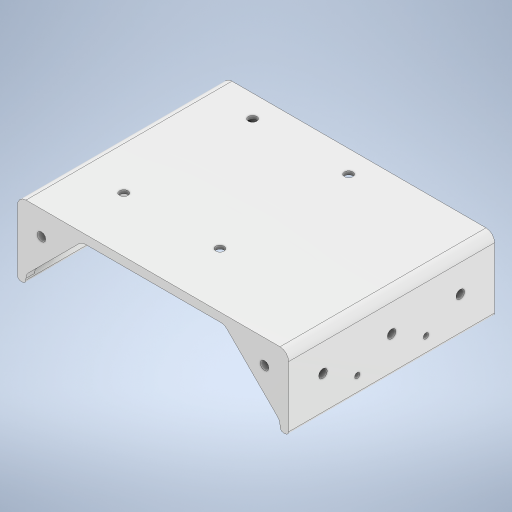
# Autodesk Inventor part: BP_BOX-Side-120-2
Saved by Autodesk Inventor 2024.3 (Build 283343000, 343)
## iProperties
Created: 2025-10-30
Part Number: BP_BOX-Side-120-2
Material: ABS プラスチック
Document SubType Name: Modeling
Designer: 佐藤智貴
Density: 1.06 g/cm^3
Appearance: 滑らか - 白
Mass: 64.4893 g
Surface Area: 354.929 cm^2
Volume: 60.8389 cm^3
Author: 佐藤智貴
Autodesk Inventor part; units mm, degrees
ref_plane "YZ Plane" through (0, 0, 0) normal (1, 0, 0) x (0, 1, 0)
ref_plane "XZ Plane" through (0, 0, 0) normal (0, 1, 0) x (-1, 0, 0)
ref_plane "XY Plane" through (0, 0, 0) normal (0, 0, 1) x (1, 0, 0)
sketch "スケッチ1" plane through (0, 0, 0) normal (0, 0, 1) x (1, 0, 0)
  line L0 (0, 0) -> (158, 0)
  line L1 (158, 0) -> (158, 250)
  line L2 (158, 250) -> (0, 250)
  line L3 (0, 250) -> (0, 0)
  line L4 (5, 245) -> (153, 245)
  line L5 (153, 245) -> (153, 5)
  line L6 (153, 5) -> (5, 5)
  line L7 (5, 5) -> (5, 245)
  line L8 (79, 250) -> (79, 0)
  line L9 (0, 125) -> (158, 125)
  line L10 (0, 245) -> (158, 245)
  line L11 (158, 245) -> (158, 3)
  line L12 (158, 3) -> (0, 3)
  line L13 (0, 3) -> (0, 245)
  point P0 (158, 245)
  point P1 (0, 3)
  point P2 (79, 3)
  point P3 (79, 5)
  point P4 (5, 125)
  point P5 (153, 125)
  point P6 (79, 245)
  point P7 (79, 245)
  point P8 (79, 125)
  point P9 (0, 3)
  dimension "d0" = 158
  dimension "d1" = 250
  dimension "d2" = 5
  dimension "d73" = 5
  constraints: 28 end point, 6 parallel, 4 midpoint, 3 perpendicular, 2 horizontal, 2 point on line, 3 other
  measures "d0" distance of L1.end L2.end
  measures "d1" distance between parallel lines of L0 L2
  measures "d2" distance between parallel lines of L2 L4
  measures "d73" distance between parallel lines of L2 L10
extrude "押し出し1" add sketch "スケッチ1" along normal blind 120 contours L3 L2 L8 L4 L10 | L10 L4 L8 L2 L1
sketch "スケッチ5" plane through (0, 0, 0) normal (0, 0, -1) x (-1, 0, 0)
  line L0 (0, 250) -> (0, 0) projected
  line L1 (0, 250) -> (-50, 250)
  line L2 (-50, 250) -> (-50, 200)
  line L3 (-50, 200) -> (0, 200)
  line L4 (0, 200) -> (0, 250)
  line L5 (-50, 250) -> (0, 200)
  line L6 (-46.2132, 253.7868) -> (3.7868, 203.7868)
  line L7 (0, 0) -> (-158, 0) projected
  line L8 (0, 125) -> (-79, 125)
  line L9 (-79, 125) -> (-79, 0)
  line L10 (-79, 0) -> (0, 0)
  line L11 (0, 0) -> (0, 125)
  line L12 (-46.2132, -3.7868) -> (3.7868, 46.2132)
  line L13 (-111.7868, 253.7868) -> (-161.7868, 203.7868)
  line L14 (-111.7868, -3.7868) -> (-161.7868, 46.2132)
  line L15 (0, 0) -> (-50, 0)
  line L16 (0, 50) -> (0, 0)
  line L17 (-158, 250) -> (-158, 0)
  line L18 (-158, 0) -> (0, 0)
  line L19 (-158, 250) -> (-108, 250)
  point P0 (0, 42.4264)
  point P1 (-42.4264, 0)
  point P2 (-158, 42.4264)
  point P3 (-115.5736, 0)
  point P4 (-42.4264, 250)
  point P5 (0, 207.5736)
  point P6 (-115.5736, 250)
  point P7 (-158, 207.5736)
  dimension "d29" = 50
  dimension "d30" = 50
  dimension "d31" = 30
  constraints: 36 end point, 12 symmetric about line, 5 parallel, 2 horizontal, 2 midpoint, 2 perpendicular
  measures "d29" distance of L2.end L3.end
  measures "d30" distance of L1.end L2.end
  measures "d31" distance from line of L0.start L6
extrude "押し出し3" add sketch "スケッチ5" against normal blind 5 contours L0 L6 L1 | L13 L17 L19
sketch "スケッチ6" plane through (0, 0, 120) normal (0, 0, 1) x (1, 0, 0)
  line L0 (0, 0) -> (50, 0)
  line L1 (50, 0) -> (50, 50)
  line L2 (50, 50) -> (0, 50)
  line L3 (0, 50) -> (0, 0)
  line L4 (50, 0) -> (0, 50)
  line L5 (46.2132, -3.7868) -> (-3.7868, 46.2132)
  line L6 (0, 250) -> (0, 0) projected
  line L7 (158, 250) -> (0, 250) projected
  line L8 (0, 125) -> (79, 125)
  line L9 (79, 125) -> (79, 250)
  line L10 (79, 250) -> (0, 250)
  line L11 (0, 250) -> (0, 125)
  line L12 (0, 250) -> (50, 250)
  line L13 (0, 200) -> (0, 250)
  line L14 (46.2132, 253.7868) -> (-3.7868, 203.7868)
  line L15 (158, 0) -> (108, 0)
  line L16 (158, 50) -> (158, 0)
  line L17 (111.7868, -3.7868) -> (161.7868, 46.2132)
  line L18 (158, 250) -> (158, 0)
  line L19 (158, 250) -> (108, 250)
  line L20 (111.7868, 253.7868) -> (161.7868, 203.7868)
  point P0 (158, 42.4264)
  point P1 (115.5736, 0)
  point P2 (158, 207.5736)
  point P3 (115.5736, 250)
  point P4 (0, 207.5736)
  point P5 (42.4264, 250)
  point P6 (42.4264, 0)
  point P7 (0, 42.4264)
  dimension "d34" = 50
  dimension "d35" = 50
  dimension "d37" = 30
  constraints: 38 end point, 14 symmetric about line, 5 parallel, 2 horizontal, 2 midpoint, 2 perpendicular
  measures "d34" distance of L1.end L2.end
  measures "d35" distance of L0.end L1.end
  measures "d37" distance from line of L5 L0.start
extrude "押し出し4" add sketch "スケッチ6" against normal blind 5 contours L6 L7 L14 | L18 L20 L7
sketch "スケッチ7" plane through (0, 0, 0) normal (0, 0, -1) x (-1, 0, 0)
  line L0 (0, 0) -> (-158, 0) projected
  line L1 (0, 124.7294) -> (-79, 124.7294)
  line L2 (-79, 124.7294) -> (-79, 0)
  line L3 (-79, 0) -> (0, 0)
  line L4 (0, 0) -> (0, 124.7294)
  line L5 (0, 250) -> (0, 0) projected
  line L6 (-158, 250) -> (0, 250) projected
  point P0 (-14, 236)
  point P1 (-14, 13.4587)
  point P2 (-144, 236)
  point P3 (-144, 13.4587)
  point P4 (0, 207.5736)
  dimension "d70" = 130
  dimension "d71" = 14
  dimension "d72" = 14
  constraints: 8 end point, 3 symmetric about line, 2 parallel, 1 horizontal, 1 midpoint, 1 perpendicular
  measures "d70" distance of point (-144, 236) point (-14, 236)
  measures "d71" distance from line of L5 point (-14, 236)
  measures "d72" distance from line of L6 point (-144, 236)
hole "穴2" at (14, 236, 0) at (14, 13.4587, 0) at (144, 236, 0) at (144, 13.4587, 0) direction (0, 0, 1) diameter 5 end through all
sketch "スケッチ8" plane through (158, 250, 120) normal (1, 0, 0) x (0, 0, -1)
  line L0 (120, 0) -> (0, 0) projected
  line L1 (120, -42.4264) -> (115, -42.4264) projected
  line L2 (0, 0) -> (120, 0)
  line L3 (120, 0) -> (120, -42.4264)
  line L4 (120, -42.4264) -> (0, -42.4264)
  line L5 (0, -42.4264) -> (0, 0)
  point P0 (120, -250)
  constraints: 8 end point, 2 parallel, 1 horizontal, 1 perpendicular
extrude "押し出し5" add sketch "スケッチ8" against normal blind 5
sketch "スケッチ9" plane through (0, 250, 0) normal (-1, 0, 0) x (0, 0, 1)
  line L0 (120, 0) -> (120, -42.4264) projected
  line L1 (0, 0) -> (0, -250) projected
  line L2 (120, 0) -> (0, 0)
  line L3 (0, 0) -> (0, -42.4264)
  line L4 (0, -42.4264) -> (120, -42.4264)
  line L5 (120, -42.4264) -> (120, 0)
  point P0 (120, -42.4264)
  point P1 (60, -250)
  constraints: 8 end point, 2 parallel, 1 horizontal, 1 perpendicular, 1 other
extrude "押し出し6" add sketch "スケッチ9" against normal blind 5
fillet "フィレット4" radius 5 12 edges at (0, 250, 60) (158, 250, 60) (120.5736, 245, 117.5) (120.5736, 245, 2.5) (153, 245, 60) (5, 245, 60) (37.4264, 245, 117.5) (37.4264, 245, 2.5) (153, 212.5736, 2.5) (153, 212.5736, 117.5) (5, 212.5736, 2.5) (5, 212.5736, 117.5)
fillet "フィレット6" radius 2 4 edges at (153, 207.5736, 60) (0, 207.5736, 60) (5, 207.5736, 60) (158, 207.5736, 60)
sketch "スケッチ12" plane through (37.4264, 245, 0) normal (0, -1, 0) x (1, 0, 0)
  line L0 (-27.4264, 5) -> (2.0711, 5) projected
  line L1 (2.0711, 0) -> (81.0761, 0) projected
  line L2 (81.0761, 5) -> (110.5736, 5) projected
  line L3 (110.5736, 115) -> (81.0761, 115) projected
  line L4 (2.0711, 120) -> (81.0761, 120) projected
  line L5 (2.0711, 115) -> (-27.4264, 115) projected
  line L6 (78.1472, 115) -> (78.1472, 110)
  line L7 (78.1472, 110) -> (108.5736, 110)
  line L8 (108.5736, 110) -> (108.5736, 10)
  line L9 (108.5736, 10) -> (76.1819, 10)
  line L10 (76.1819, 10) -> (76.1819, 5)
  line L11 (76.1819, 5) -> (3.0347, 5)
  line L12 (3.0347, 5) -> (3.0347, 10)
  line L13 (3.0347, 10) -> (-25.4264, 10)
  line L14 (-25.4264, 10) -> (-25.4264, 110)
  line L15 (-25.4264, 110) -> (3.0347, 110)
  line L16 (3.0347, 110) -> (3.0347, 115)
  line L17 (3.0347, 115) -> (78.1472, 115)
  line L18 (2.0711, 0) -> (2.0711, 5) projected
  line L19 (81.0761, 5) -> (81.0761, 0) projected
  line L20 (110.5736, 115) -> (110.5736, 5) projected
  line L21 (81.0761, 120) -> (81.0761, 115) projected
  line L22 (2.0711, 115) -> (2.0711, 120) projected
  line L23 (-27.4264, 5) -> (-27.4264, 115) projected
  line L24 (115.5736, 120) -> (115.5736, 0) projected
  line L25 (-32.4264, 0) -> (-32.4264, 120) projected
  point P0 (-37.4264, 0)
  dimension "d76" = 5
  dimension "d81" = 7
  dimension "d82" = 5
  dimension "d84" = 7
  dimension "d85" = 5
  dimension "d86" = 5
  constraints: 24 end point
  measures "d76" distance between parallel lines of L4 L17
  measures "d81" distance between parallel lines of L24 L8
  measures "d82" distance between parallel lines of L25 L23
  measures "d84" distance between parallel lines of L25 L14
  measures "d85" distance between parallel lines of L15 L5
  measures "d86" distance between parallel lines of L0 L13
extrude "押し出し8" cut sketch "スケッチ12" against normal blind 3 contours L6 L7 L8 L9 L10 L11 L12 L13 L14 L15 L16 L17
fillet "フィレット7" radius 2 12 edges at (146, 246.5, 10) (146, 246.5, 110) (115.5736, 246.5, 110) (113.6083, 246.5, 10) (115.5736, 246.5, 115) (113.6083, 246.5, 5) (40.4611, 246.5, 5) (40.4611, 246.5, 10) (12, 246.5, 10) (40.4611, 246.5, 115) (40.4611, 246.5, 110) (12, 246.5, 110)
sketch "スケッチ13" plane through (0, 245, 0) normal (-1, 0, 0) x (0, 0, 1)
  circle A0 centre (10, -16) radius 2.5 projected
  line L0 (10, -16) -> (115, -16)
  line L1 (115, -34.4975) -> (115, -5) projected
  line L2 (120, 5) -> (0, 5) projected
  circle A1 centre (100, -16) radius 2.5
  circle A2 centre (60, -16) radius 2.5
  circle A3 centre (20, -16) radius 2.5
  line L3 (120, 0) -> (120, -35.4264) projected
  line L4 (0, 0) -> (0, -35.4264) projected
  circle A4 centre (10, -27) radius 1.6 projected
  line L5 (10, -27) -> (115, -27)
  circle A5 centre (40, -27) radius 1.6
  circle A6 centre (80, -27) radius 1.6
  point P0 (0, -245)
  point P1 (0, -17.7132)
  dimension "d87" = 21
  dimension "d88" = 20
  dimension "d89" = 5
  dimension "d90" = 5
  dimension "d91" = 5
  dimension "d92" = 20
  dimension "d93" = 40
  dimension "d94" = 3.2
  dimension "d95" = 3.2
  dimension "d96" = 40
  dimension "d97" = 20
  constraints: 7 point on line, 5 centre point, 4 end point, 2 horizontal, 1 midpoint
  measures "d87" distance between parallel lines of L2 L0
  measures "d88" distance from line of L3 A1.centre
  measures "d89" diameter of A1
  measures "d90" diameter of A2
  measures "d91" diameter of A3
  measures "d92" horizontal distance of point (0, -17.713) A3.centre
  measures "d93" distance of A3.centre A2.centre
  measures "d94" diameter of A6
  measures "d95" diameter of A5
  measures "d96" distance of A6.centre A5.centre
  measures "d97" horizontal distance of A6.centre A2.centre
extrude "押し出し9" cut sketch "スケッチ13" against normal through all contours A3 L0 | L0 A3 | A2 L0 | L0 A2 | A1 L0 | L0 A1 | A5 L5 | L5 A5 | A6 L5 | L5 A6
sketch "スケッチ14" plane through (5, 250, 0) normal (0, 1, 0) x (1, 0, 0)
  line L0 (148, -120) -> (0, -120) projected
  line L1 (-5, 0) -> (-5, -120) projected
  line L2 (148, 0) -> (0, 0) projected
  point P0 (81, -88)
  point P1 (25, -88)
  point P2 (25, -13)
  point P3 (81, -13)
  dimension "d102" = 56
  dimension "d103" = 30
  dimension "d104" = 75
  dimension "d105" = 75
  dimension "d106" = 56
  dimension "d107" = 30
  dimension "d115" = 13
  dimension "d116" = 13
  dimension "d117" = 32
  measures "d102" distance of point (81, -88) point (25, -88)
  measures "d103" distance from line of L1 point (25, -88)
  measures "d104" distance of point (25, -88) point (25, -13)
  measures "d105" distance of point (81, -88) point (81, -13)
  measures "d106" distance of point (81, -13) point (25, -13)
  measures "d107" distance from line of L1 point (25, -13)
  measures "d115" distance from line of L2 point (25, -13)
  measures "d116" distance from line of L2 point (81, -13)
  measures "d117" distance from line of L0 point (81, -88)
hole "穴3" at (86, 250, 88) at (30, 250, 88) at (30, 250, 13) at (86, 250, 13) direction (0, -1, 0) diameter 5 end through all
equation "\"d35\" = d34"
equation "\"d85\" = d76"
equation "\"d90\" = d89"
equation "\"d91\" = d90"
equation "\"d92\" = d88"
equation "\"d95\" = d94"
equation "\"d96\" = d93"
equation "\"d97\" = 0.5 * d96"
equation "\"d105\" = d104"
equation "\"d106\" = d102"
equation "\"d107\" = d103"
equation "\"d116\" = d115"
